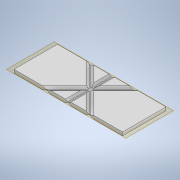
# Autodesk Inventor part: test_hangle_org_2
Saved by Autodesk Inventor 2020 (Build 240168000, 168)
## iProperties
Created: 2021-04-08
Part Number: test_hangle_org_2
Material: Generic
Document SubType Name: Modeling
Designer: Shuang Peng
Density: 1 g/cm^3
Appearance: Default
Author: Shuang Peng
Autodesk Inventor part; units mm, degrees
ref_plane "YZ Plane" through (0, 0, 0) normal (1, 0, 0) x (0, 1, 0)
ref_plane "XZ Plane" through (0, 0, 0) normal (0, 1, 0) x (-1, 0, 0)
ref_plane "XY Plane" through (0, 0, 0) normal (0, 0, 1) x (1, 0, 0)
sketch "Sketch1" plane through (0, 0, 0) normal (0, 1, 0) x (-1, 0, 0)
  line L0 (0, 0) -> (50, 0)
  line L1 (50, 0) -> (50, -20)
  line L2 (50, -20) -> (0, -20)
  line L3 (0, -20) -> (0, 0)
  line L4 (25, 0) -> (25, -20)
  line L5 (25, -20) -> (35, -20)
  line L6 (25, 0) -> (35, 0)
  line L7 (25, 0) -> (15, 0)
  line L8 (25, -20) -> (15, -20)
  line L9 (15, -20) -> (25, -10)
  line L10 (25, -10) -> (15, 0)
  line L11 (25, -10) -> (35, -20)
  line L12 (25, -10) -> (35, 0)
  line L13 (25.25, 2.5) -> (24.75, 2.5)
  line L14 (24.75, 2.5) -> (24.75, -22.5)
  line L15 (24.75, -22.5) -> (25.25, -22.5)
  line L16 (25.25, -22.5) -> (25.25, 2.5)
  line L17 (25.25, 2.5) -> (24.75, -22.5) construction
  line L18 (24.75, 2.5) -> (25.25, -22.5) construction
  line L19 (7.499107, 7.854446) -> (7.145554, 7.500893)
  line L20 (7.145554, 7.500893) -> (42.500893, -27.854446)
  line L21 (42.500893, -27.854446) -> (42.854446, -27.500893)
  line L22 (42.854446, -27.500893) -> (7.499107, 7.854446)
  line L23 (7.499107, 7.854446) -> (42.500893, -27.854446) construction
  line L24 (7.145554, 7.500893) -> (42.854446, -27.500893) construction
  line L25 (42.854446, 7.500893) -> (42.500893, 7.854446)
  line L26 (42.500893, 7.854446) -> (7.145554, -27.500893)
  line L27 (7.145554, -27.500893) -> (7.499107, -27.854446)
  line L28 (7.499107, -27.854446) -> (42.854446, 7.500893)
  line L29 (42.854446, 7.500893) -> (7.145554, -27.500893) construction
  line L30 (42.500893, 7.854446) -> (7.499107, -27.854446) construction
  point P0 (14.646447, -20)
  point P1 (24.646447, -10)
  point P2 (14.646447, 0)
  point P3 (24.75, -10.603553)
  point P4 (15.353553, -20)
  point P5 (24.75, -20)
  point P6 (34.646447, -20)
  point P7 (25.25, -10.603553)
  point P8 (25.25, -20)
  point P9 (15.353553, 0)
  point P10 (24.75, -9.396447)
  point P11 (24.75, 0)
  point P12 (25.25, -9.396447)
  point P13 (34.646447, 0)
  point P14 (25.25, 0)
  point P15 (35.353553, 0)
  point P16 (25.353553, -10)
  point P17 (35.353553, -20)
  dimension "d0" = 50
  dimension "d1" = 20
  dimension "d2" = 10
  dimension "d3" = 10
  dimension "d4" = 10
  dimension "d5" = 10
  dimension "d6" = 0.5
  dimension "d7" = 25
  dimension "d8" = 0.5
  dimension "d9" = 50
  dimension "d10" = 0.5
  dimension "d11" = 50
  constraints: 62 end point, 9 midpoint, 8 parallel, 6 perpendicular, 4 point on line, 2 horizontal
  measures "d0" distance of L1.end L2.end
  measures "d1" distance of L0.end L1.end
  measures "d2" distance of L4.end L5.end
  measures "d3" distance of L4.start L6.end
  measures "d4" distance of L4.start L7.end
  measures "d5" distance of L4.end L8.end
  measures "d6" distance of L13.start L13.end
  measures "d7" distance of L14.end L13.end
  measures "d8" distance of L19.start L19.end
  measures "d9" distance of L20.end L19.end
  measures "d10" distance of L25.start L25.end
  measures "d11" distance of L26.end L25.end
extrude "Extrusion1" add sketch "Sketch1" along normal blind 1.5 contours L0 L20 L26 L2 L3 | L0 L14 L22 | L28 L14 L2 | L0 L26 L16 | L20 L2 L16 | L28 L0 L1 L2 L22
ref_plane "Work Plane1" through (0, 0.75, 0) normal (0, 1, 0) x (1, 0, 0)
sketch "Sketch2" plane through (0, 0.75, 0) normal (0, 1, 0) x (1, 0, 0)
  line L0 (-50, 20) -> (-50, 0)
  line L1 (-35.353553, 20) -> (-50, 20)
  line L2 (-25.353553, 10) -> (-35.353553, 20)
  line L3 (-35.353553, 0) -> (-25.353553, 10)
  line L4 (-50, 0) -> (-35.353553, 0)
  line L5 (-25.25, 9.396447) -> (-34.646447, 0)
  line L6 (-25.25, 0) -> (-25.25, 9.396447)
  line L7 (-34.646447, 0) -> (-25.25, 0)
  line L8 (-24.75, 9.396447) -> (-24.75, 0)
  line L9 (-15.353553, 0) -> (-24.75, 9.396447)
  line L10 (-24.75, 0) -> (-15.353553, 0)
  line L11 (-24.646447, 10) -> (-14.646447, 0)
  line L12 (-14.646447, 20) -> (-24.646447, 10)
  line L13 (0, 20) -> (-14.646447, 20)
  line L14 (0, 0) -> (0, 20)
  line L15 (-14.646447, 0) -> (0, 0)
  line L16 (-15.353553, 20) -> (-24.75, 20)
  line L17 (-24.75, 10.603553) -> (-15.353553, 20)
  line L18 (-24.75, 20) -> (-24.75, 10.603553)
  line L19 (-25.25, 20) -> (-34.646447, 20)
  line L20 (-25.25, 10.603553) -> (-25.25, 20)
  line L21 (-34.646447, 20) -> (-25.25, 10.603553)
  line L22 (-50, 0) -> (-35.353553, 0)
  line L23 (-50, 0) -> (0, 0)
  line L24 (-50, 20) -> (0, 20)
  constraints: 4 end point, 1 collinear, 1 parallel
extrude "Extrusion2" add sketch "Sketch2" along normal mid plane 0.29 contours L24 L21 L20 L18 L17 L12 L11 L23 L9 L8 L6 L5 L3 L2
chamfer "Chamfer1" distance 1 distance2 0.605 1 edges at (-30.3536, 1.5, -5) measured on face at (-30.7071, 1.5, -5.3536)
chamfer "Chamfer2" distance 1 distance2 0.605 1 edges at (-29.9482, 1.5, -4.6982) measured on face at (-29.5947, 1.5, -4.3447)
chamfer "Chamfer3" distance 1 distance2 0.605 1 edges at (-30.7071, 1.5, -15.3535) measured on face at (-31.0606, 1.5, -15)
chamfer "Chamfer4" distance 1 distance2 0.605 1 edges at (-29.9482, 1.5, -15.3018) measured on face at (-29.5947, 1.5, -15.6553)
chamfer "Chamfer5" distance 1 distance2 0.605 1 edges at (-25.25, 1.5, -16.0088) measured on face at (-25.75, 1.5, -16.0088)
chamfer "Chamfer6" distance 1 distance2 0.605 1 edges at (-24.75, 1.5, -15.3018) measured on face at (-24.25, 1.5, -15.3018)
chamfer "Chamfer7" distance 1 distance2 0.605 1 edges at (-25.25, 1.5, -3.9912) measured on face at (-25.75, 1.5, -3.9912)
chamfer "Chamfer8" distance 1 distance2 0.605 1 edges at (-24.75, 1.5, -4.6982) measured on face at (-24.25, 1.5, -4.6982)
chamfer "Chamfer9" distance 1 distance2 0.605 1 edges at (-19.5518, 1.5, -4.1983) measured on face at (-19.9054, 1.5, -3.8447)
chamfer "Chamfer10" distance 1 distance2 0.605 1 edges at (-19.6464, 1.5, -5) measured on face at (-19.2929, 1.5, -5.3536)
chamfer "Chamfer11" distance 1 distance2 0.605 1 edges at (-19.5518, 1.5, -15.8017) measured on face at (-19.9054, 1.5, -16.1553)
chamfer "Chamfer12" distance 1 distance2 0.605 1 edges at (-19.2929, 1.5, -15.3535) measured on face at (-18.9394, 1.5, -15)
chamfer "Chamfer13" distance 0.605 distance2 1 1 edges at (-29.9482, 0, -15.3018) measured on face at (-29.9482, 0.1, -15.3018)
chamfer "Chamfer14" distance 0.605 distance2 1 1 edges at (-30.3536, 0, -15) measured on face at (-30.3536, 0.1, -15)
chamfer "Chamfer15" distance 0.605 distance2 1 1 edges at (-25.25, 0, -16.0088) measured on face at (-25.25, 0.1, -16.0088)
chamfer "Chamfer16" distance 0.605 distance2 1 1 edges at (-24.75, 0, -15.3018) measured on face at (-24.75, 0.1, -15.3018)
chamfer "Chamfer17" distance 0.605 distance2 1 1 edges at (-19.5518, 0, -15.8017) measured on face at (-19.5518, 0.1, -15.8017)
chamfer "Chamfer18" distance 0.605 distance2 1 1 edges at (-19.6464, 0, -15) measured on face at (-19.6464, 0.1, -15)
chamfer "Chamfer19" distance 0.605 distance2 1 1 edges at (-19.2929, 0, -4.6465) measured on face at (-19.2929, 0.1, -4.6465)
chamfer "Chamfer20" distance 0.605 distance2 1 1 edges at (-20.0518, 0, -4.6982) measured on face at (-20.0518, 0.1, -4.6982)
chamfer "Chamfer21" distance 0.605 distance2 1 1 edges at (-24.75, 0, -3.9912) measured on face at (-24.75, 0.1, -3.9912)
chamfer "Chamfer22" distance 0.605 distance2 1 1 edges at (-25.25, 0, -4.6982) measured on face at (-25.25, 0.1, -4.6982)
chamfer "Chamfer23" distance 0.605 distance2 1 1 edges at (-30.4482, 0, -4.1983) measured on face at (-30.4482, 0.1, -4.1983)
chamfer "Chamfer24" distance 0.605 distance2 1 1 edges at (-30.7071, 0, -4.6465) measured on face at (-30.7071, 0.1, -4.6465)
body "Solid1"
